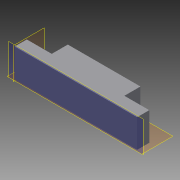
# Autodesk Inventor part: cabinet
Saved by Autodesk Inventor 2015 (Build 190159000, 159)
## iProperties
Created: 2015-10-18
Part Number: cabinet
Material: 一般
Document SubType Name: Modeling
Designer: omae
Density: 1 g/cm^3
Appearance: 既定
Author: omae
Autodesk Inventor part; units mm, degrees
sketch "スケッチ1" plane through (0, 0, 0) normal (1, 0, 0) x (0, 1, 0)
  line L0 (0, 0) -> (325.8, 0)
  line L1 (325.8, 0) -> (325.8, 754)
  line L2 (325.8, 754) -> (0, 754)
  line L3 (0, 754) -> (0, 0)
  dimension "d0" = 325.8
  dimension "d1" = 754
  constraints: 8 end point, 2 parallel, 1 horizontal, 1 perpendicular
  measures "d0" distance of L2.end L1.end
  measures "d1" distance of L1.end L0.end
extrude "押し出し1" add sketch "スケッチ1" along normal blind 665
sketch "スケッチ2" plane through (665, 0, 0) normal (1, 0, 0) x (0, 0, -1)
  line L0 (0, 0) -> (-754, 0)
  line L1 (-754, 0) -> (-754, 755)
  line L2 (-754, 755) -> (0, 755)
  line L3 (0, 755) -> (0, 0)
  dimension "d4" = 754
  dimension "d5" = 755
  constraints: 8 end point, 2 parallel, 1 horizontal, 1 perpendicular
  measures "d4" distance of L1.end L2.end
  measures "d5" distance of L0.end L1.end
extrude "押し出し2" add sketch "スケッチ2" along normal blind 1939
sketch "スケッチ3" plane through (2604, 0, 0) normal (1, 0, 0) x (0, 0, -1)
  line L0 (0, 0) -> (-754, 0)
  line L1 (-754, 0) -> (-754, 325.8)
  line L2 (-754, 325.8) -> (0, 325.8)
  line L3 (0, 325.8) -> (0, 0)
  dimension "d8" = 754
  dimension "d9" = 325.8
  constraints: 8 end point, 2 parallel, 1 horizontal, 1 perpendicular
  measures "d8" distance of L1.end L2.end
  measures "d9" distance of L0.end L1.end
extrude "押し出し3" add sketch "スケッチ3" along normal blind 665
